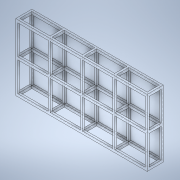
# Autodesk Inventor part: CustomAquariumsStand
Saved by Autodesk Inventor 2022 (Build 260153000, 153)
## iProperties
Created: 2021-06-25
Part Number: CustomAquariumsStand
Material: Generic
Document SubType Name: Modeling
Designer: jamieson-bl
Density: 1 g/cm^3
Appearance: Default
Author: jamieson-bl
Autodesk Inventor part; units mm, degrees
ref_plane "YZ Plane" through (0, 0, 0) normal (1, 0, 0) x (0, 1, 0)
ref_plane "XZ Plane" through (0, 0, 0) normal (0, 1, 0) x (-1, 0, 0)
ref_plane "XY Plane" through (0, 0, 0) normal (0, 0, 1) x (1, 0, 0)
sketch "Sketch1" plane through (0, 0, 0) normal (0, 0, 1) x (1, 0, 0)
  line L0 (1219.2, -609.6) -> (-1219.2, -609.6)
  line L1 (-1219.2, -609.6) -> (-1219.2, 609.6)
  line L2 (-1219.2, 609.6) -> (1219.2, 609.6)
  line L3 (1219.2, 609.6) -> (1219.2, -609.6)
  line L4 (1219.2, -609.6) -> (-1219.2, 609.6) construction
  line L5 (-1219.2, -609.6) -> (1219.2, 609.6) construction
  point P0 (0, 0)
  dimension "d0" = 2438.4
  dimension "d1" = 1219.2
  constraints: 12 end point, 2 midpoint, 2 parallel, 1 horizontal, 1 perpendicular
  measures "d0" distance of L1.end L2.end
  measures "d1" distance of L0.end L1.end
extrude "Extrusion1" add sketch "Sketch1" along normal blind 19.05
sketch "Sketch2" plane through (0, 0, 19.05) normal (0, 0, 1) x (1, 0, 0)
  line L0 (-1238.25, -628.65) -> (1238.25, -628.65)
  line L1 (1238.25, -628.65) -> (1238.25, 628.65)
  line L2 (1238.25, 628.65) -> (-1238.25, 628.65)
  line L3 (-1238.25, 628.65) -> (-1238.25, -628.65)
  line L4 (-1238.25, -628.65) -> (1238.25, 628.65) construction
  line L5 (1238.25, -628.65) -> (-1238.25, 628.65) construction
  line L6 (1200.15, -577.85) -> (-1200.15, -577.85)
  line L7 (-1200.15, -577.85) -> (-1200.15, 577.85)
  line L8 (-1200.15, 577.85) -> (1200.15, 577.85)
  line L9 (1200.15, 577.85) -> (1200.15, -577.85)
  line L10 (1200.15, -577.85) -> (-1200.15, 577.85) construction
  line L11 (-1200.15, -577.85) -> (1200.15, 577.85) construction
  point P0 (0, 0)
  dimension "d4" = 2476.5
  dimension "d5" = 1257.3
  dimension "d6" = 2400.3
  dimension "d7" = 1155.7
  constraints: 24 end point, 4 midpoint, 4 parallel, 2 horizontal, 2 perpendicular
  measures "d4" distance of L2.end L1.end
  measures "d5" distance of L1.end L0.end
  measures "d6" distance of L7.end L8.end
  measures "d7" distance of L6.end L7.end
extrude "Extrusion2" add sketch "Sketch2" along normal blind 38.1
sketch "Sketch4" plane through (0, 0, 19.05) normal (0, 0, 1) x (1, 0, 0)
  line L0 (-1200.15, 577.85) -> (-1200.15, -577.85) projected
  line L1 (-1238.25, 628.65) -> (-1200.15, 628.65)
  line L2 (-1200.15, 628.65) -> (-1200.15, 577.85)
  line L3 (-1200.15, 577.85) -> (-1238.25, 577.85)
  line L4 (-1238.25, 577.85) -> (-1238.25, 628.65)
  line L5 (-590.55, 577.85) -> (-628.65, 577.85)
  line L6 (-590.55, 628.65) -> (-590.55, 577.85)
  line L7 (-628.65, 628.65) -> (-590.55, 628.65)
  line L8 (-628.65, 577.85) -> (-628.65, 628.65)
  line L9 (19.05, 577.85) -> (-19.05, 577.85)
  line L10 (19.05, 628.65) -> (19.05, 577.85)
  line L11 (-19.05, 628.65) -> (19.05, 628.65)
  line L12 (-19.05, 577.85) -> (-19.05, 628.65)
  line L13 (628.65, 577.85) -> (590.55, 577.85)
  line L14 (628.65, 628.65) -> (628.65, 577.85)
  line L15 (590.55, 628.65) -> (628.65, 628.65)
  line L16 (590.55, 577.85) -> (590.55, 628.65)
  line L17 (1238.25, 577.85) -> (1200.15, 577.85)
  line L18 (1238.25, 628.65) -> (1238.25, 577.85)
  line L19 (1200.15, 628.65) -> (1238.25, 628.65)
  line L20 (1200.15, 577.85) -> (1200.15, 628.65)
  line L21 (-1200.15, -25.4) -> (-1238.25, -25.4)
  line L22 (-1200.15, 25.4) -> (-1200.15, -25.4)
  line L23 (-1238.25, 25.4) -> (-1200.15, 25.4)
  line L24 (-1238.25, -25.4) -> (-1238.25, 25.4)
  line L25 (-590.55, -25.4) -> (-628.65, -25.4)
  line L26 (-590.55, 25.4) -> (-590.55, -25.4)
  line L27 (-628.65, 25.4) -> (-590.55, 25.4)
  line L28 (-628.65, -25.4) -> (-628.65, 25.4)
  line L29 (19.05, -25.4) -> (-19.05, -25.4)
  line L30 (19.05, 25.4) -> (19.05, -25.4)
  line L31 (-19.05, 25.4) -> (19.05, 25.4)
  line L32 (-19.05, -25.4) -> (-19.05, 25.4)
  line L33 (628.65, -25.4) -> (590.55, -25.4)
  line L34 (628.65, 25.4) -> (628.65, -25.4)
  line L35 (590.55, 25.4) -> (628.65, 25.4)
  line L36 (590.55, -25.4) -> (590.55, 25.4)
  line L37 (1238.25, -25.4) -> (1200.15, -25.4)
  line L38 (1238.25, 25.4) -> (1238.25, -25.4)
  line L39 (1200.15, 25.4) -> (1238.25, 25.4)
  line L40 (1200.15, -25.4) -> (1200.15, 25.4)
  line L41 (-1200.15, -628.65) -> (-1238.25, -628.65)
  line L42 (-1200.15, -577.85) -> (-1200.15, -628.65)
  line L43 (-1238.25, -577.85) -> (-1200.15, -577.85)
  line L44 (-1238.25, -628.65) -> (-1238.25, -577.85)
  line L45 (-590.55, -628.65) -> (-628.65, -628.65)
  line L46 (-590.55, -577.85) -> (-590.55, -628.65)
  line L47 (-628.65, -577.85) -> (-590.55, -577.85)
  line L48 (-628.65, -628.65) -> (-628.65, -577.85)
  line L49 (19.05, -628.65) -> (-19.05, -628.65)
  line L50 (19.05, -577.85) -> (19.05, -628.65)
  line L51 (-19.05, -577.85) -> (19.05, -577.85)
  line L52 (-19.05, -628.65) -> (-19.05, -577.85)
  line L53 (628.65, -628.65) -> (590.55, -628.65)
  line L54 (628.65, -577.85) -> (628.65, -628.65)
  line L55 (590.55, -577.85) -> (628.65, -577.85)
  line L56 (590.55, -628.65) -> (590.55, -577.85)
  line L57 (1238.25, -628.65) -> (1200.15, -628.65)
  line L58 (1238.25, -577.85) -> (1238.25, -628.65)
  line L59 (1200.15, -577.85) -> (1238.25, -577.85)
  line L60 (1200.15, -628.65) -> (1200.15, -577.85)
  point P0 (0, 0)
  dimension "d35" = 609.6
  dimension "d38" = 603.25
  constraints: 120 end point, 2 collinear, 2 horizontal, 2 parallel, 1 perpendicular, 1 vertical, 110 other
  measures "d35" distance of L0.start L5.start
  measures "d38" distance of L0.start L21.start
extrude "Extrusion3" add sketch "Sketch4" along normal blind 304.8
sketch "Sketch5" plane through (0, 0, 19.05) normal (0, 0, 1) x (1, 0, 0)
  line L0 (-1238.25, -25.4) -> (-1200.15, -25.4) projected
  line L1 (-628.65, -25.4) -> (-628.65, 25.4) projected
  line L2 (-1200.15, -25.4) -> (-628.65, -25.4)
  line L3 (-628.65, -25.4) -> (-628.65, 25.4)
  line L4 (-628.65, 25.4) -> (-1200.15, 25.4)
  line L5 (-1200.15, 25.4) -> (-1200.15, -25.4)
  line L6 (-590.55, -25.4) -> (-590.55, 25.4) projected
  line L7 (-628.65, 577.85) -> (-590.55, 577.85) projected
  line L8 (-590.55, 25.4) -> (-628.65, 25.4)
  line L9 (-628.65, 25.4) -> (-628.65, 577.85)
  line L10 (-628.65, 577.85) -> (-590.55, 577.85)
  line L11 (-590.55, 577.85) -> (-590.55, 25.4)
  line L12 (-590.55, 25.4) -> (-590.55, -25.4)
  line L13 (-19.05, 25.4) -> (-590.55, 25.4)
  line L14 (-590.55, -25.4) -> (-19.05, -25.4)
  line L15 (-19.05, -25.4) -> (-19.05, 25.4)
  line L16 (19.05, 25.4) -> (-19.05, 25.4)
  line L17 (-19.05, 25.4) -> (-19.05, 577.85)
  line L18 (19.05, 577.85) -> (19.05, 25.4)
  line L19 (-19.05, 577.85) -> (19.05, 577.85)
  line L20 (19.05, 25.4) -> (19.05, -25.4)
  line L21 (590.55, 25.4) -> (19.05, 25.4)
  line L22 (19.05, -25.4) -> (590.55, -25.4)
  line L23 (590.55, -25.4) -> (590.55, 25.4)
  line L24 (628.65, 25.4) -> (590.55, 25.4)
  line L25 (590.55, 25.4) -> (590.55, 577.85)
  line L26 (628.65, 577.85) -> (628.65, 25.4)
  line L27 (590.55, 577.85) -> (628.65, 577.85)
  line L28 (628.65, 25.4) -> (628.65, -25.4)
  line L29 (1200.15, 25.4) -> (628.65, 25.4)
  line L30 (628.65, -25.4) -> (1200.15, -25.4)
  line L31 (1200.15, -25.4) -> (1200.15, 25.4)
  line L32 (1238.25, 25.4) -> (1200.15, 25.4)
  line L33 (1200.15, 25.4) -> (1200.15, 577.85)
  line L34 (1238.25, 577.85) -> (1238.25, 25.4)
  line L35 (1200.15, 577.85) -> (1238.25, 577.85)
  line L36 (-1200.15, -577.85) -> (-1200.15, -628.65)
  line L37 (-628.65, -577.85) -> (-1200.15, -577.85)
  line L38 (-1200.15, -628.65) -> (-628.65, -628.65)
  line L39 (-628.65, -628.65) -> (-628.65, -577.85)
  line L40 (-590.55, -577.85) -> (-628.65, -577.85)
  line L41 (-628.65, -577.85) -> (-628.65, -25.4)
  line L42 (-590.55, -25.4) -> (-590.55, -577.85)
  line L43 (-628.65, -25.4) -> (-590.55, -25.4)
  line L44 (-590.55, -577.85) -> (-590.55, -628.65)
  line L45 (-19.05, -577.85) -> (-590.55, -577.85)
  line L46 (-590.55, -628.65) -> (-19.05, -628.65)
  line L47 (-19.05, -628.65) -> (-19.05, -577.85)
  line L48 (19.05, -577.85) -> (-19.05, -577.85)
  line L49 (-19.05, -577.85) -> (-19.05, -25.4)
  line L50 (19.05, -25.4) -> (19.05, -577.85)
  line L51 (-19.05, -25.4) -> (19.05, -25.4)
  line L52 (19.05, -577.85) -> (19.05, -628.65)
  line L53 (590.55, -577.85) -> (19.05, -577.85)
  line L54 (19.05, -628.65) -> (590.55, -628.65)
  line L55 (590.55, -628.65) -> (590.55, -577.85)
  line L56 (628.65, -577.85) -> (590.55, -577.85)
  line L57 (590.55, -577.85) -> (590.55, -25.4)
  line L58 (628.65, -25.4) -> (628.65, -577.85)
  line L59 (590.55, -25.4) -> (628.65, -25.4)
  line L60 (628.65, -577.85) -> (628.65, -628.65)
  line L61 (1200.15, -577.85) -> (628.65, -577.85)
  line L62 (628.65, -628.65) -> (1200.15, -628.65)
  line L63 (1200.15, -628.65) -> (1200.15, -577.85)
  line L64 (1238.25, -577.85) -> (1200.15, -577.85)
  line L65 (1200.15, -577.85) -> (1200.15, -25.4)
  line L66 (1238.25, -25.4) -> (1238.25, -577.85)
  line L67 (1200.15, -25.4) -> (1238.25, -25.4)
  point P0 (0, 0)
  dimension "d43" = 609.6
  dimension "d46" = 603.25
  constraints: 128 end point, 4 parallel, 3 horizontal, 2 collinear, 2 perpendicular, 1 vertical, 110 other
  measures "d43" distance of L4.end L12.start
  measures "d46" distance of L4.end L36.start
extrude "Extrusion4" add sketch "Sketch5" along normal blind 38.1 contours L2 L5 L4 L1 | L43 L42 L40 L41 | L9 L7 L11 L8 | L6 L13 L15 L14 | L51 L50 L48 L49 | L17 L19 L18 L16 | L20 L21 L23 L22 | L59 L58 L56 L57 | L25 L27 L26 L24 | L28 L29 L31 L30
pattern_linear "Rectangular Pattern1" count 2 spacing 266.7 along (0, 0, 1) of "Extrusion4", "Extrusion2"
body "Solid1"
